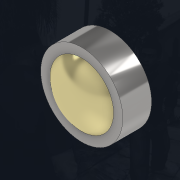
# Autodesk Inventor part: Button1
Saved by Autodesk Inventor 2021 (Build 250183000, 183)
## iProperties
Created: 2021-01-08
Part Number: Button1
Material: Generic
Document SubType Name: Modeling
Designer: Alex
Density: 1 g/cm^3
Appearance: Default
Author: Alex
Autodesk Inventor part; units mm, degrees
ref_plane "YZ Plane" through (0, 0, 0) normal (1, 0, 0) x (0, 1, 0)
ref_plane "XZ Plane" through (0, 0, 0) normal (0, 1, 0) x (-1, 0, 0)
ref_plane "XY Plane" through (0, 0, 0) normal (0, 0, 1) x (1, 0, 0)
sketch "Sketch1" plane through (0, 0, 0) normal (0, 0, 1) x (1, 0, 0)
  line L0 (14, 0) -> (-14, 0)
  line L1 (0, 0) -> (0, 47)
  line L2 (0, 47) -> (0, 57)
  circle A0 centre (0, 57) radius 10
  circle A1 centre (0, 57) radius 8.5
  dimension "d0" = 47
  dimension "d1" = 10
  dimension "d2" = 1.5
  constraints: 6 end point, 2 vertical, 1 centre point, 1 coincident, 1 midpoint, 1 vertical alignment, 2 other
  measures "d0" distance of L1.start L1.end
  measures "d1" distance of L1.end L2.end
extrude "Extrusion1" add sketch "Sketch1" along normal blind 7
sketch "Sketch2" plane through (0, 57, 0) normal (0, 0, -1) x (-1, 0, 0)
  circle A0 centre (0, 0) radius 7.75
  point P0 (0, -57)
  dimension "d5" = 15.5
  constraints: 1 centre point
  measures "d5" diameter of A0
extrude "Extrusion2" add sketch "Sketch2" against normal up to surface (7 mm away)
sketch "Sketch3" plane through (0, 57, 0) normal (0, 0, -1) x (-1, 0, 0)
  circle A0 centre (0, 0) radius 7.75 projected
  circle A1 centre (0, 0) radius 10
  point P0 (0, -57)
  constraints: 1 centre point, 1 coincident
extrude "Extrusion3" add sketch "Sketch3" against normal blind 4 contours A0 | A1
sketch "Sketch4" plane through (0, 0, 0) normal (1, 0, 0) x (0, 1, 0)
  line L0 (57, 0) -> (57, 7)
  line L1 (48.5, 7) -> (65.5, 7) projected
  line L2 (57, 7) -> (57, 10)
  line L3 (64.75, 4) -> (64.75, 7) projected
  line L4 (49.25, 4) -> (49.25, 7) projected
  arc A0 (64.75, 7) -> (49.25, 7) centre (57, -1.5104) ccw
  point P0 (0, 0)
  dimension "d10" = 3
  constraints: 4 end point, 4 point on line, 3 point on circle, 1 centre point, 1 midpoint, 1 vertical
  measures "d10" distance of L0.end L2.end
revolve "Revolution1" add sketch "Sketch4" angle 360 about axis through (0, 57, 7) along (0, 0, 1) picked at (52.6027, 7.5441) contours A0 L2 L1
sketch "Sketch5" plane through (0, 57, 7) normal (0, 0, 1) x (1, 0, 0)
  circle A0 centre (0, 0) radius 7.75
  circle A1 centre (0, 0) radius 8.5
  point P0 (0, -57)
  constraints: 2 centre point, 1 coincident
extrude "Extrusion4" add sketch "Sketch5" against normal up to surface (7 mm away)
body "Solid1"
